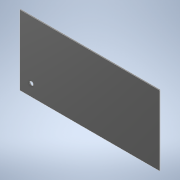
# Autodesk Inventor part: 後ろカバー
Saved by Autodesk Inventor 2022 (Build 260153000, 153)
## iProperties
Created: 2022-11-07
Part Number: 後ろカバー
Material: 一般
Document SubType Name: Modeling
Designer: tdn82
Density: 1 g/cm^3
Appearance: 既定
Author: tdn82
Autodesk Inventor part; units mm, degrees
ref_plane "YZ Plane" through (0, 0, 0) normal (1, 0, 0) x (0, 1, 0)
ref_plane "XZ Plane" through (0, 0, 0) normal (0, 1, 0) x (-1, 0, 0)
ref_plane "XY Plane" through (0, 0, 0) normal (0, 0, 1) x (1, 0, 0)
sketch "スケッチ1" plane through (0, 0, 0) normal (0, 0, 1) x (1, 0, 0)
  line L0 (0, 0) -> (360, 0)
  line L1 (360, 0) -> (360, -180)
  line L2 (360, -180) -> (0, -180)
  line L3 (0, -180) -> (0, 0)
  dimension "d0" = 360
  dimension "d1" = 180
  constraints: 8 end point, 2 parallel, 1 horizontal, 1 perpendicular
  measures "d0" distance of L0.start L0.end
  measures "d1" distance of L2.end L0.start
extrude "押し出し1" add sketch "スケッチ1" along normal blind 2
sketch "スケッチ2" plane through (0, 0, 2) normal (0, 0, 1) x (1, 0, 0)
  line L0 (0, -180) -> (360, -180) projected
  line L1 (360, -180) -> (360, 0) projected
  line L2 (0, 0) -> (0, -180) projected
  point P0 (30, -150)
  dimension "d4" = 30
  dimension "d13" = 30
  measures "d4" distance from line of L0 point (30, -150)
  measures "d13" distance from line of L2 point (30, -150)
hole "穴1" at (30, -150, 2) direction (0, 0, -1) diameter 10 end through all
